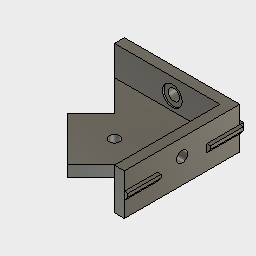
CornerTrussBrace (Autodesk Fusion 360 design; units mm, degrees)
Autodesk Fusion 360 part; units mm, degrees
sketch "Sketch1" plane through (0, 0, 0) normal (0, 0, 1) x (1, 0, 0) in component "corner truss brace (1)"
  line L0 (82.6456, 31.4944) -> (82.6456, -3.4575)
  line L1 (82.6456, -3.4575) -> (79.6456, -3.4575)
  line L2 (79.6456, -3.4575) -> (70.444, 5.744)
  line L3 (70.444, 5.744) -> (63.3358, -1.3642)
  line L4 (63.3358, -1.3642) -> (49.9008, 12.0708)
  line L5 (49.9008, 12.0708) -> (57.0112, 19.1813)
  line L6 (57.0112, 19.1813) -> (47.6981, 28.4944)
  line L7 (47.6981, 28.4944) -> (47.6981, 31.4944)
  line L8 (47.6981, 31.4944) -> (82.6456, 31.4944)
  line L9 (79.6456, -3.4575) -> (79.6456, 28.4944)
  line L10 (79.6456, 28.4944) -> (47.6981, 28.4944)
  circle A0 centre (63.7271, 12.4621) radius 1.6
  arc A1 (57.0112, 19.1813) -> (70.444, 5.744) centre (41484.8849, 41420.1849) ccw construction
  dimension "d162" = 45
  dimension "d163" = 3
  dimension "d164" = 3
  dimension "d165" = 3.2
  dimension "d169" = 19
  dimension "d170" = 9.5
  constraint vertical L0
  constraint perpendicular L0 L1
  constraint perpendicular L3 L4
  constraint perpendicular L4 L5
  constraint vertical L7
  constraint perpendicular L1 L9
  constraint horizontal L8
  constraint parallel L8 L10
  constraint parallel L2 L4
  constraint parallel L4 L6
  constraint tangent L2 A1
  constraint midpoint A1
  measures "d162" angle of L0 L4
  measures "d163" distance of L8 L10
  measures "d164" distance of L0 L9
  measures "d165" diameter of A0
extrude "Extrude1" add sketch "Sketch1" along normal blind 12.5 contours L0 L1 L7 L8 L9 L10 makes body 1 in component "corner truss brace (1)"
extrude "Extrude2" add sketch "Sketch1" along normal blind 3.5 contours L2 L3 L4 L5 L6 L9 L10 bodies 1 in component "corner truss brace (1)"
sketch "Sketch2" plane through (0, 28.4944, 0) normal (0, -1, 0) x (1, 0, 0) in component "corner truss brace (1)"
  line L0 (47.6981, 3.5) -> (79.6456, 3.5)
  line L1 (79.6456, 3.5) -> (79.6456, 12.5)
  line L2 (79.6456, 12.5) -> (47.6981, 12.5)
  line L3 (47.6981, 12.5) -> (47.6981, 3.5)
  circle A0 centre (65.1981, 7.5) radius 1.7
  circle A1 centre (65.1981, 7.5) radius 3
  dimension "d175" = 3.4
  dimension "d178" = 1.3
  dimension "d179" = 17.5
  dimension "d180" = 5
  constraint midpoint L3
  measures "d175" diameter of A0
  measures "d180" distance of L2
sketch "Sketch3" plane through (79.6456, 0, 0) normal (-1, 0, 0) x (0, -1, 0) in component "corner truss brace (1)"
  line L0 (-28.4944, 3.5) -> (3.4575, 3.5)
  line L1 (3.4575, 3.5) -> (3.4575, 12.5)
  line L2 (3.4575, 12.5) -> (-28.4944, 12.5)
  line L3 (-28.4944, 12.5) -> (-28.4944, 3.5)
  circle A0 centre (-14.0425, 7.5) radius 1.7
  circle A1 centre (-14.0425, 7.5) radius 3
  dimension "d176" = 3.4
  dimension "d177" = 1.3
  dimension "d181" = 17.5
  dimension "d182" = 5
  constraint midpoint L1
  measures "d176" diameter of A0
  measures "d182" distance of L2
extrude "Extrude3" cut sketch "Sketch2" against normal blind 0.5 contours A1 bodies 1 in component "corner truss brace (1)"
extrude "Extrude4" cut sketch "Sketch2" against normal up to surface (3 mm away) contours A0 bodies 1 in component "corner truss brace (1)"
extrude "Extrude5" cut sketch "Sketch3" against normal blind 0.5 contours A1 bodies 1 in component "corner truss brace (1)"
extrude "Extrude6" cut sketch "Sketch3" against normal up to surface (3 mm away) contours A0 bodies 1 in component "corner truss brace (1)"
sketch "Sketch5" plane through (0, -3.4575, 0) normal (0, -1, 0) x (1, 0, 0) in component "corner truss brace (1)"
  line L0 (79.6456, 0) -> (82.6456, 0)
  line L1 (82.6456, 0) -> (82.6456, 12.5)
  line L2 (82.6456, 12.5) -> (79.6456, 12.5)
  line L3 (79.6456, 12.5) -> (79.6456, 3.5)
  line L4 (79.6456, 3.5) -> (79.6456, 0)
  line L5 (82.6456, 7.1528) -> (82.6456, 4.7528)
  line L6 (82.6456, 7.1528) -> (83.7456, 7.1528)
  line L7 (83.7456, 7.1528) -> (83.7456, 6.1528)
  line L8 (83.7456, 6.1528) -> (82.6456, 4.7528)
  dimension "d189" = 2.4
  dimension "d190" = 1.1
  dimension "d191" = 1
  constraint coincident L1
  constraint parallel L1 L5
  constraint perpendicular L5 L6
extrude "Extrude7" add sketch "Sketch5" against normal blind 10 separate body contours L1 L5 L6 L7 L8 makes body 2 in component "corner truss brace (1)"
copy_body "CopyPasteBodies1" bodies 2 makes body 3 in component "corner truss brace (1)"
move_body "MoveBody1" bodies 3 to x (1, 0, 0) y (0, 1, 0) z (0, 0, 1) at (0, 25, 0) in component "corner truss brace (1)"
copy_body "CopyPasteBodies2" bodies 2 makes body 4 in component "corner truss brace (1)"
move_body "MoveBody2" bodies 4 to x (0, 1, 0) y (-1, 0, 0) z (0, 0, 1) at (79.1881, -51.1032, 0) in component "corner truss brace (1)"
copy_body "CopyPasteBodies3" bodies 4 makes body 5 in component "corner truss brace (1)"
move_body "MoveBody3" bodies 5 to x (1, 0, 0) y (0, 1, 0) z (0, 0, 1) at (-25, 0, 0) in component "corner truss brace (1)"
component "corner truss brace (1)" placed x (1, 0, 0) y (0, 1, 0) z (0, 0, 1) at (0, 0, 0)
